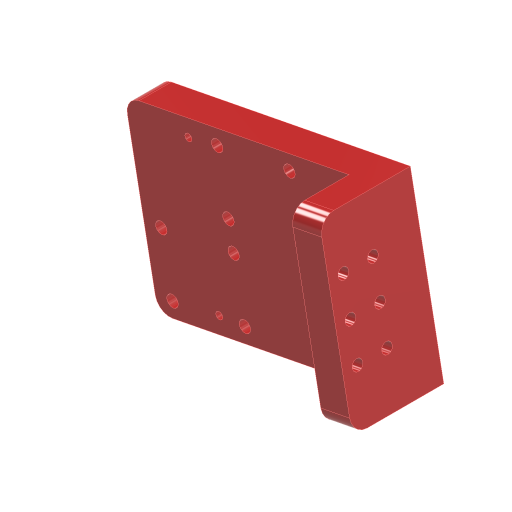
# Autodesk Inventor part: Uchwyt_arduino
Saved by Autodesk Inventor 2024.3 (Build 283343000, 343)
## iProperties
Created: 2025-06-24
Part Number: Uchwyt_arduino
Material: PET Plastic
Document SubType Name: Modeling
Designer: MPA
Density: 1.541 g/cm^3
Appearance: Red
Author: MPA
Autodesk Inventor part; units mm, degrees
ref_plane "YZ Plane" through (0, 0, 0) normal (1, 0, 0) x (0, 1, 0)
ref_plane "XZ Plane" through (0, 0, 0) normal (0, 1, 0) x (-1, 0, 0)
ref_plane "XY Plane" through (0, 0, 0) normal (0, 0, 1) x (1, 0, 0)
sketch "Sketch1" plane through (0, 0, 0) normal (0, 0, 1) x (1, 0, 0)
  circle A0 centre (-46.9442, -24.6808) radius 1.05 construction
  circle A1 centre (0, 0) radius 1.05 construction
  circle A2 centre (-5.3474, 27.4235) radius 1.05 construction
  circle A3 centre (-57.4271, 22.4441) radius 1.05 construction
  line L0 (-60.4322, -29.8783) -> (1.8719, -17.7295) construction
  line L1 (-7.8098, 34.6865) -> (-70.6332, 22.4365) construction
  line L2 (-71.419, 21.27) -> (-61.6027, -29.0717) construction
  line L3 (2.8951, -1.7497) -> (-3.3696, 30.3784) construction
  line L4 (-61.3651, -30.0949) -> (5.9074, -16.8925) construction
  line L5 (5.9074, -16.8925) -> (-4.3581, 35.4149) construction
  line L6 (-4.3581, 35.4149) -> (-71.6306, 22.2125) construction
  line L7 (-71.6306, 22.2125) -> (-61.3651, -30.0949) construction
  line L8 (-61.3651, -30.0949) -> (-4.3581, 35.4149) construction
  line L9 (5.9074, -16.8925) -> (-71.6306, 22.2125) construction
  line L10 (-70.6332, 22.4365) -> (-71.6306, 22.2125) construction
  line L11 (-71.6306, 22.2125) -> (-71.419, 21.27) construction
  line L12 (-61.6027, -29.0717) -> (-61.3651, -30.0949) construction
  line L13 (-61.3651, -30.0949) -> (-60.4322, -29.8783) construction
  line L14 (-72.6327, -35.3485) -> (18.2757, -17.6221)
  line L15 (18.2757, -17.6221) -> (6.9095, 40.6685)
  line L16 (6.9095, 40.6685) -> (-83.9989, 22.9421)
  line L17 (-83.9989, 22.9421) -> (-72.6327, -35.3485)
  line L18 (-72.6327, -35.3485) -> (6.9095, 40.6685) construction
  line L19 (18.2757, -17.6221) -> (-83.9989, 22.9421) construction
  point P0 (0, 0)
  point P1 (-32.8616, 2.66)
  dimension "d0" = 3
  dimension "d1" = 12
  constraints: 32 end point, 8 parallel, 4 midpoint, 4 perpendicular, 1 point on line
  measures "d0" distance from line of L16 L5.end
  measures "d1" distance from line of L15 L4.end
extrude "Extrusion1" add sketch "Sketch1" along normal blind 11
sketch "Sketch2" plane through (0, 0, 0) normal (0, 0, -1) x (-1, 0, 0)
  point P0 (0, 0)
  point P1 (5.3474, 27.4235)
  point P2 (57.4271, 22.4441)
  point P3 (46.9442, -24.6808)
  point P4 (0, 0)
hole "Hole1" at (-5.3474, 27.4235, 0) at (-57.4271, 22.4441, 0) at (-46.9442, -24.6808, 0) at (0, 0, 0) direction (0, 0, 1) diameter 2.4 end through all clearance for "Countersunk Flat Head Screw DIN EN ISO 2009" size "M2" standard "DIN"
sketch "Sketch3" plane through (0, 0, 0) normal (0, 0, -1) x (-1, 0, 0)
  circle A0 centre (57.4271, 22.4441) radius 1.2 projected
  circle A1 centre (46.9442, -24.6808) radius 1.2 projected
  circle A2 centre (0, 0) radius 1.2 projected
  circle A3 centre (5.3474, 27.4235) radius 1.2 projected
  point P0 (0, 0)
hole "Hole2" at (-57.4271, 22.4441, 0) at (-46.9442, -24.6808, 0) at (0, 0, 0) at (-5.3474, 27.4235, 0) direction (0, 0, 1) diameter 3.6 depth 3
sketch "Sketch4" plane through (0, 0, 11) normal (0, 0, 1) x (1, 0, 0)
  circle A0 centre (0, 0) radius 1.2 projected
  circle A1 centre (-46.9442, -24.6808) radius 1.2 projected
  circle A2 centre (-57.4271, 22.4441) radius 1.2 projected
  circle A3 centre (-5.3474, 27.4235) radius 1.2 projected
  line L0 (18.2757, -17.6221) -> (6.9095, 40.6685) projected
  line L1 (6.9095, 40.6685) -> (-83.9989, 22.9421) projected
  line L2 (-83.9989, 22.9421) -> (-72.6327, -35.3485) projected
  line L3 (-72.6327, -35.3485) -> (18.2757, -17.6221) projected
  line L4 (-2.9056, 38.7546) -> (8.4605, -19.536)
  line L5 (8.4605, -19.536) -> (18.2757, -17.6221)
  line L6 (18.2757, -17.6221) -> (6.9095, 40.6685)
  line L7 (6.9095, 40.6685) -> (-2.9056, 38.7546)
  line L8 (-2.9056, 38.7546) -> (18.2757, -17.6221) construction
  line L9 (8.4605, -19.536) -> (6.9095, 40.6685) construction
  point P0 (0, 0)
  point P1 (7.685, 10.5663)
  point P2 (-2.9056, 38.7546)
  point P3 (8.4605, -19.536)
  dimension "d18" = 10
  constraints: 12 end point, 2 midpoint, 2 parallel, 1 perpendicular
  measures "d18" distance between parallel lines of L0 L4
extrude "Extrusion2" add sketch "Sketch4" along normal blind 20 contours L3 L4 L1 L0
sketch "Sketch5" plane through (8.4605, -19.536, 11) normal (-0.9815146, -0.1913872, 0) x (0, 0, 1)
  line L0 (0, 0) -> (0, 59.3885) projected
  line L1 (0, 0) -> (20, 0) projected
  line L2 (20, 59.3885) -> (20, 0) projected
  line L3 (0, 59.3885) -> (20, 59.3885) projected
  line L4 (15, 17.1942) -> (5, 17.1942) construction
  line L5 (5, 17.1942) -> (5, 42.1942) construction
  line L6 (5, 42.1942) -> (15, 42.1942) construction
  line L7 (15, 42.1942) -> (15, 17.1942) construction
  line L8 (15, 17.1942) -> (5, 42.1942) construction
  line L9 (5, 17.1942) -> (15, 42.1942) construction
  point P0 (-11, 20.7941)
  point P1 (10, 29.6942)
  point P2 (20, 29.6942)
  point P3 (10, 42.1942)
  point P4 (10, 59.3885)
  point P5 (15, 29.6942)
  point P6 (5, 29.6942)
  dimension "d21" = 25
  dimension "d22" = 10
  constraints: 12 end point, 7 midpoint, 4 coincident, 2 parallel, 1 horizontal, 1 horizontal alignment, 1 perpendicular, 1 vertical alignment
  measures "d21" distance of L6.end L4.start
  measures "d22" distance of L5.end L6.end
hole "Hole3" at (0.3851, 21.8782, 16) at (0.3851, 21.8782, 26) at (5.1698, -2.6596, 26) at (5.1698, -2.6596, 16) at (2.7775, 9.6093, 26) at (2.7775, 9.6093, 16) direction (0.9815146, 0.1913872, 0) diameter 3.6 end through all clearance for "Countersunk Flat Head Screw DIN EN ISO 2009" size "M3" standard "DIN"
move faces "Move1" translate (4.9076, 0.9569, 0) faces at (-80.2101, 3.5119, 3.6667)
fillet "Fillet1" radius 5 4 edges at (-79.0913, 23.8991, 5.5) (-67.7251, -34.3916, 5.5) (2.0019, 39.7116, 31) (13.3681, -18.5791, 31)
sketch "Sketch6" plane through (0, 0, 11) normal (0, 0, 1) x (1, 0, 0)
  line L0 (-1.9487, 33.8471) -> (7.5036, -14.6284) projected
  line L1 (-47.6531, 24.9351) -> (-23.1153, 29.7198) construction
  line L2 (-23.1153, 29.7198) -> (-19.2875, 10.0895) construction
  line L3 (-19.2875, 10.0895) -> (-43.8254, 5.3048) construction
  line L4 (-43.8254, 5.3048) -> (-47.6531, 24.9351) construction
  circle A0 centre (-5.3474, 27.4235) radius 1.2 projected
  line L5 (-2.9056, 38.7546) -> (-74.1837, 24.856) projected
  line L6 (-66.6207, -8.7054) -> (-42.0828, -3.9207) construction
  line L7 (-42.0828, -3.9207) -> (-38.2551, -23.551) construction
  line L8 (-38.2551, -23.551) -> (-62.7929, -28.3357) construction
  line L9 (-62.7929, -28.3357) -> (-66.6207, -8.7054) construction
  line L10 (-62.8175, -33.4346) -> (8.4605, -19.536) projected
  line L11 (-78.1343, 18.9915) -> (-68.682, -29.484) projected
  point P0 (0, 0)
  dimension "d49" = 25
  dimension "d50" = 20
  dimension "d51" = 17
  dimension "d52" = 5
  dimension "d54" = 20
  dimension "d55" = 25
  dimension "d56" = 5
  dimension "d57" = 6
  constraints: 16 end point, 8 coincident, 6 parallel, 2 perpendicular
  measures "d49" distance of L1.start L1.end
  measures "d50" distance of L1.end L2.end
  measures "d51" distance from line of L2 A0.centre
  measures "d52" distance between parallel lines of L5 L1
  measures "d54" distance of L6.end L7.end
  measures "d55" distance of L6.start L6.end
  measures "d56" distance between parallel lines of L10 L8
  measures "d57" distance between parallel lines of L11 L9
hole "Hole4" at (-47.6531, 24.9351, 11) at (-43.8254, 5.3048, 11) at (-19.2875, 10.0895, 11) at (-23.1153, 29.7198, 11) at (-66.6207, -8.7054, 11) at (-42.0828, -3.9207, 11) at (-38.2551, -23.551, 11) at (-62.7929, -28.3357, 11) direction (0, 0, -1) diameter 2.6 end through all clearance for "Countersunk Flat Head Screw DIN EN ISO 2009" size "M2" standard "DIN"
sketch "Sketch7" plane through (0, 0, 11) normal (0, 0, 1) x (1, 0, 0)
  circle A0 centre (-47.6531, 24.9351) radius 1.3 projected
  circle A1 centre (-43.8254, 5.3048) radius 1.3 projected
  circle A2 centre (-23.1153, 29.7198) radius 1.3 projected
  circle A3 centre (-19.2875, 10.0895) radius 1.3 projected
  circle A4 centre (-66.6207, -8.7054) radius 1.3 projected
  circle A5 centre (-42.0828, -3.9207) radius 1.3 projected
  circle A6 centre (-38.2551, -23.551) radius 1.3 projected
  circle A7 centre (-62.7929, -28.3357) radius 1.3 projected
  point P0 (0, 0)
hole "Hole5" at (-47.6531, 24.9351, 11) at (-43.8254, 5.3048, 11) at (-19.2875, 10.0895, 11) at (-23.1153, 29.7198, 11) at (-66.6207, -8.7054, 11) at (-42.0828, -3.9207, 11) at (-38.2551, -23.551, 11) at (-62.7929, -28.3357, 11) direction (0, 0, -1) diameter 3.9 depth 3
chamfer "Chamfer1" distance 0.6 angle 45 4 edges at (-5.3474, 26.2235, 3) (0, -1.2, 3) (-46.9442, -25.8808, 3) (-57.4271, 21.2441, 3)
equation "\"d54\" = d50"
equation "\"d55\" = d49"
equation "\"d56\" = d52"
body "Solid1"
